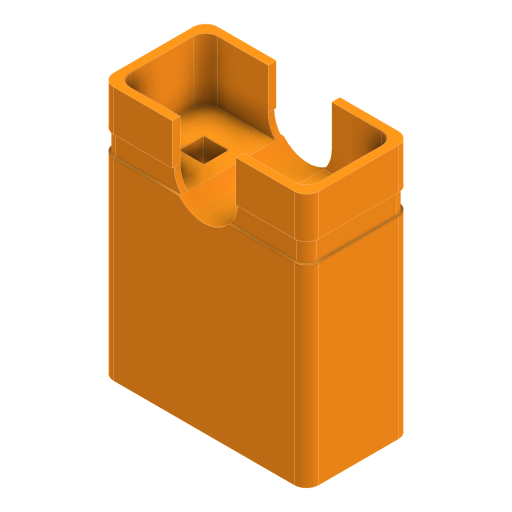
# Autodesk Inventor part: Retrigger Resetting Jumper
Saved by Autodesk Inventor 2024 (Build 280153000, 153)
## iProperties
Created: 2024-09-24
Part Number: Retrigger Resetting Jumper
Material: Generic
Document SubType Name: Modeling
Designer: Laith Al-Sadi
Density: 1 g/cm^3
Appearance: Orange
Author: Laith Al-Sadi
Autodesk Inventor part; units mm, degrees
ref_plane "YZ Plane" through (0, 0, 0) normal (1, 0, 0) x (0, 1, 0)
ref_plane "XZ Plane" through (0, 0, 0) normal (0, 1, 0) x (-1, 0, 0)
ref_plane "XY Plane" through (0, 0, 0) normal (0, 0, 1) x (1, 0, 0)
sketch "Sketch1" plane through (0, 0, 0) normal (0, 0, 1) x (1, 0, 0)
  line L0 (-2.5, 3.1) -> (2.5, 3.1)
  line L1 (2.5, 3.1) -> (2.5, -3.1)
  line L2 (2.5, -3.1) -> (-2.5, -3.1)
  line L3 (-2.5, -3.1) -> (-2.5, 3.1)
  line L4 (-2.5, 3.1) -> (2.5, -3.1) construction
  line L5 (2.5, 3.1) -> (-2.5, -3.1) construction
  line L6 (-0.775, 3.1) -> (-0.775, 2.1)
  line L7 (0.775, 3.1) -> (0.775, 2.1)
  arc A0 (-0.775, 2.1) -> (0.775, 2.1) centre (0, 2.1) ccw
  point P0 (0, 0)
  point P1 (0, 3.1)
  dimension "d0" = 6.2
  dimension "d1" = 5
  dimension "d2" = 1
  dimension "d3" = 1
  dimension "d4" = 1.55
  constraints: 16 end point, 3 midpoint, 2 parallel, 2 perpendicular, 2 point on circle, 2 point on line, 1 centre point, 1 horizontal, 1 tangent, 1 vertical, 1 vertical alignment
  measures "d0" distance of L0.end L1.end
  measures "d1" distance of L0.start L0.end
  measures "d2" distance of L6.start L6.end
  measures "d3" distance of L7.start L7.end
  measures "d4" distance of L7.start L6.start
extrude "Extrusion1" add sketch "Sketch1" along normal blind 2.54 contours L0 L6 A0 L7 L1 L2 L3
sketch "Sketch2" plane through (-2.5, 3.1, 0) normal (0, 1, 0) x (1, 0, 0)
  line L0 (0.2, -2.34) -> (4.8, -2.34)
  line L1 (4.8, -2.34) -> (4.8, -0.2)
  line L2 (4.8, -0.2) -> (0.2, -0.2)
  line L3 (0.2, -0.2) -> (0.2, -2.34)
  line L4 (0.2, -2.34) -> (4.8, -0.2) construction
  line L5 (4.8, -2.34) -> (0.2, -0.2) construction
  line L6 (0, 0) -> (0, -2.54) projected
  line L7 (1.725, 0) -> (0, 0) projected
  point P0 (2.5, 0)
  point P1 (2.5, -1.27)
  point P2 (0, -1.27)
  point P3 (0.8625, 0)
  dimension "d7" = 0.2
  dimension "d8" = 0.2
  constraints: 12 end point, 4 midpoint, 2 parallel, 1 horizontal, 1 horizontal alignment, 1 perpendicular, 1 vertical alignment
  measures "d7" distance between parallel lines of L6 L3
  measures "d8" distance from line of point (0.862, 0) L2
extrude "Extrusion2" cut sketch "Sketch2" against normal blind 1.5
sketch "Sketch3" plane through (-2.5, 1.6, 0) normal (0, 1, 0) x (1, 0, 0)
  line L0 (0.93, -0.97) -> (1.53, -0.97)
  line L1 (1.53, -0.97) -> (1.53, -1.57)
  line L2 (1.53, -1.57) -> (0.93, -1.57)
  line L3 (0.93, -1.57) -> (0.93, -0.97)
  line L4 (0.93, -0.97) -> (1.53, -1.57) construction
  line L5 (1.53, -0.97) -> (0.93, -1.57) construction
  line L6 (3.47, -0.97) -> (4.07, -0.97)
  line L7 (4.07, -0.97) -> (4.07, -1.57)
  line L8 (4.07, -1.57) -> (3.47, -1.57)
  line L9 (3.47, -1.57) -> (3.47, -0.97)
  line L10 (3.47, -0.97) -> (4.07, -1.57) construction
  line L11 (4.07, -0.97) -> (3.47, -1.57) construction
  line L12 (5, 0) -> (5, -2.54) projected
  point P0 (2.5, 0)
  point P1 (1.23, -1.27)
  point P2 (3.77, -1.27)
  point P3 (5, -1.27)
  dimension "d11" = 0.6
  dimension "d12" = 0.6
  dimension "d13" = 0.6
  dimension "d14" = 0.6
  dimension "d15" = 2.54
  dimension "d16" = 1.27
  constraints: 24 end point, 5 midpoint, 4 parallel, 2 horizontal, 2 perpendicular, 1 horizontal alignment, 1 point on line
  measures "d11" distance of L0.start L0.end
  measures "d12" distance of L0.end L1.end
  measures "d13" distance of L6.start L6.end
  measures "d14" distance of L8.end L6.start
  measures "d15" distance of point (1.23, -1.27) point (3.77, -1.27)
  measures "d16" horizontal distance of point (2.5, 0) point (3.77, -1.27)
extrude "Extrusion3" cut sketch "Sketch3" against normal up to surface (4.7 mm away)
fillet "Fillet1" radius 0.3 8 edges at (-2.5, 0, 2.54) (-2.5, 0, 0) (2.5, 0, 2.54) (2.5, 0, 0) (2.3, 2.35, 0.2) (2.3, 2.35, 2.34) (-2.3, 2.35, 0.2) (-2.3, 2.35, 2.34)
sketch "Sketch4" plane through (-2.5, 1.6, 0) normal (0, 1, 0) x (1, 0, 0)
  line L0 (1.725, 0) -> (0.3, 0) projected
  arc A0 (0.3, 0) -> (0, -0.3) centre (0.3, -0.3) ccw projected
  line L1 (0, -0.3) -> (0, -2.24) projected
  arc A1 (0, -2.24) -> (0.3, -2.54) centre (0.3, -2.24) ccw projected
  line L2 (1.725, -2.54) -> (0.3, -2.54) projected
  line L3 (3.275, -2.54) -> (1.725, -2.54) projected
  line L4 (4.7, -2.54) -> (3.275, -2.54) projected
  arc A2 (4.7, -2.54) -> (5, -2.24) centre (4.7, -2.24) ccw projected
  line L5 (5, -0.3) -> (5, -2.24) projected
  arc A3 (5, -0.3) -> (4.7, 0) centre (4.7, -0.3) ccw projected
  line L6 (4.7, 0) -> (3.275, 0) projected
  line L7 (3.275, 0) -> (1.725, 0) projected
  arc A4 (0.05, -2.24) -> (0.3, -2.49) centre (0.3, -2.24) ccw
  line L8 (0.05, -2.24) -> (0.05, -0.3)
  arc A5 (0.3, -0.05) -> (0.05, -0.3) centre (0.3, -0.3) ccw
  line L9 (0.3, -0.05) -> (1.725, -0.05)
  line L10 (1.725, -0.05) -> (3.275, -0.05)
  line L11 (3.275, -0.05) -> (4.7, -0.05)
  arc A6 (4.95, -0.3) -> (4.7, -0.05) centre (4.7, -0.3) ccw
  line L12 (4.95, -0.3) -> (4.95, -2.24)
  arc A7 (4.7, -2.49) -> (4.95, -2.24) centre (4.7, -2.24) ccw
  line L13 (4.7, -2.49) -> (3.275, -2.49)
  line L14 (3.275, -2.49) -> (1.725, -2.49)
  line L15 (1.725, -2.49) -> (0.3, -2.49)
  point P0 (2.5, 0)
  dimension "d20" = 0.05
  constraints: 16 end point, 8 point on circle, 4 centre point, 11 other
  measures "d20" distance between parallel lines of L2 L15
extrude "Extrusion4" cut sketch "Sketch4" along normal blind 0.5
equation "\"d3\" = d2"
equation "\"d8\" = d7"
equation "\"d12\" = d11"
equation "\"d13\" = d11"
equation "\"d14\" = d11"
equation "\"d16\" = 0.5 * d15"
body "Solid1"
